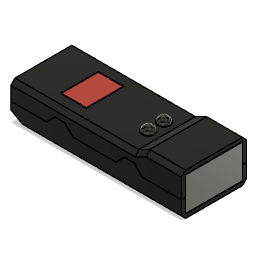
Case-USBtinyISP (Autodesk Fusion 360 design; units mm, degrees)
Autodesk Fusion 360 part; units mm, degrees
note: some values were not read from the file. Chosen so that the rebuilt part matches the saved one: which face or edge a step refers to; which pieces of a blend or face edit are solid. Set by a fixed rule: which sketch regions a step uses.
sketch "Skizze1" plane through (0, 0, 0) normal (0, 1, 0) x (1, 0, 0)
  line L0 (1, 0) -> (35.6, 0)
  line L1 (35.6, 0) -> (35.6, -15.2)
  line L2 (35.6, -15.2) -> (1, -15.2)
  line L3 (0, -14.2) -> (0, -1)
  arc A0 (1, 0) -> (0, -1) centre (1, -1) ccw
  arc A1 (0, -14.2) -> (1, -15.2) centre (1, -14.2) ccw
  line L4 (8.04, -3.725) -> (-1.46, -3.725)
  line L5 (-1.46, -3.725) -> (-1.46, -11.475)
  line L6 (-1.46, -11.475) -> (8.04, -11.475)
  line L7 (8.04, -11.475) -> (8.04, -3.725)
  line L8 (8.04, -3.725) -> (-1.46, -11.475) construction
  line L9 (-1.46, -3.725) -> (8.04, -11.475) construction
  line L10 (35.6, -7.6) -> (40.1, -7.6) construction
  line L11 (35.6, 0.02) -> (44.6, 0.02)
  line L12 (44.6, 0.02) -> (44.6, -15.22)
  line L13 (44.6, -15.22) -> (35.6, -15.22)
  line L14 (35.6, -15.22) -> (35.6, 0.02)
  line L15 (35.6, 0.02) -> (44.6, -15.22) construction
  line L16 (44.6, 0.02) -> (35.6, -15.22) construction
  line L17 (0, -7.6) -> (12, -7.6) construction
  line L18 (15.35, -2.65) -> (8.65, -2.65)
  line L19 (8.65, -2.65) -> (8.65, -12.55)
  line L20 (8.65, -12.55) -> (15.35, -12.55)
  line L21 (15.35, -12.55) -> (15.35, -2.65)
  line L22 (15.35, -2.65) -> (8.65, -12.55) construction
  line L23 (8.65, -2.65) -> (15.35, -12.55) construction
  line L24 (0, -7.6) -> (29.1, -7.6) construction
  line L25 (29.1, -7.6) -> (29.1, -5.5) construction
  line L26 (29.1, -7.6) -> (29.1, -9.7) construction
  line L27 (29.5, -6.1) -> (28.7, -6.1)
  line L28 (28.7, -6.1) -> (28.7, -4.9)
  line L29 (28.7, -4.9) -> (29.5, -4.9)
  line L30 (29.5, -4.9) -> (29.5, -6.1)
  line L31 (29.5, -6.1) -> (28.7, -4.9) construction
  line L32 (28.7, -6.1) -> (29.5, -4.9) construction
  line L33 (29.5, -10.3) -> (28.7, -10.3)
  line L34 (28.7, -10.3) -> (28.7, -9.1)
  line L35 (28.7, -9.1) -> (29.5, -9.1)
  line L36 (29.5, -9.1) -> (29.5, -10.3)
  line L37 (29.5, -10.3) -> (28.7, -9.1) construction
  line L38 (28.7, -10.3) -> (29.5, -9.1) construction
  point P0 (0, -15.2)
  point P1 (3.29, -7.6)
  point P2 (40.1, -7.6)
  point P3 (12, -7.6)
  point P4 (29.1, -5.5)
  point P5 (29.1, -9.7)
  dimension "d4" = 35.6
  dimension "d5" = 15.2
  dimension "d6" = 1
  dimension "d7" = 1
  dimension "d14" = 9.5
  dimension "d15" = 7.75
  dimension "d21" = 4.5
  dimension "d22" = 15.24
  dimension "d23" = 9
  dimension "d28" = 12
  dimension "d29" = 6.7
  dimension "d30" = 9.9
  dimension "d143" = 29.1
  dimension "d144" = 2.1
  dimension "d145" = 2.1
  dimension "d146" = 1.2
  dimension "d147" = 0.8
  dimension "d148" = 1.2
  dimension "d149" = 0.8
  dimension "d261" = 3.29
  constraint horizontal L0
  constraint vertical L1
  constraint horizontal L2
  constraint vertical L3
  constraint coincident origin L3
  constraint coincident origin L0
  constraint tangent L3 A0
  constraint tangent L0 A0
  constraint coincident P0 L2
  constraint coincident P0 L3
  constraint tangent L2 A1
  constraint tangent L3 A1
  constraint midpoint L3 L17.start
  constraint perpendicular L4 L5
  constraint parallel L4 L6
  constraint parallel L5 L7
  constraint horizontal L4
  constraint coincident L8 P1
  constraint coincident L9 P1
  constraint midpoint L1 L10.start
  constraint horizontal L10
  constraint perpendicular L11 L12
  constraint parallel L11 L13
  constraint parallel L12 L14
  constraint horizontal L11
  constraint coincident L15 P2
  constraint coincident L16 P2
  constraint coincident P2 L10.end
  constraint perpendicular L18 L19
  constraint parallel L18 L20
  constraint parallel L19 L21
  constraint horizontal L18
  constraint coincident L22 P3
  constraint coincident L23 P3
  constraint coincident P3 L17.end
  constraint horizontal L17
  constraint horizontal L24
  constraint vertical L26
  constraint vertical L25
  constraint perpendicular L27 L28
  constraint parallel L27 L29
  constraint parallel L28 L30
  constraint horizontal L27
  constraint coincident L31 P4
  constraint coincident L32 P4
  constraint coincident P4 L25.end
  constraint perpendicular L33 L34
  constraint parallel L33 L35
  constraint parallel L34 L36
  constraint horizontal L33
  constraint coincident L37 P5
  constraint coincident L38 P5
  constraint coincident P5 L26.end
  constraint coincident P1 L17
  measures "d4" distance of origin L0.end
  measures "d5" distance of origin P0
  measures "d6" radius of A0
  measures "d7" radius of A1
  measures "d14" distance of L5.end L6.end
  measures "d15" distance of L4.end L5.end
  measures "d21" distance of L10.start P2
  measures "d22" distance of L11.end L12.end
  measures "d23" distance of L12.end L13.end
  measures "d28" distance of L17.start P3
  measures "d29" distance of L19.end L20.end
  measures "d30" distance of L18.end L19.end
  measures "d143" distance of L17.start L24.end
  measures "d144" distance of L24.end P4
  measures "d145" distance of L24.end P5
  measures "d146" distance of L27.end L28.end
  measures "d147" distance of L28.end L29.end
  measures "d148" distance of L33.end L34.end
  measures "d149" distance of L34.end L35.end
  measures "d261" distance of L17.start P1
sketch "Skizze2" plane through (0, 0, 0) normal (0, 1, 0) x (1, 0, 0)
  line L0 (15.45, -12.65) -> (8.55, -12.65)
  line L1 (8.55, -12.65) -> (8.55, -2.55)
  line L2 (8.55, -2.55) -> (15.45, -2.55)
  line L3 (15.45, -2.55) -> (15.45, -12.65)
  line L4 (15.45, -12.65) -> (8.55, -2.55) construction
  line L5 (8.55, -12.65) -> (15.45, -2.55) construction
  line L6 (0, 0) -> (-0.1, 0) construction
  line L7 (-0.1, 0) -> (-0.1, 0.1) construction
  line L8 (1, 0.1) -> (44.6, 0.1)
  line L9 (44.6, 0.1) -> (44.6, -15.3)
  line L10 (44.6, -15.3) -> (1, -15.3)
  line L11 (-0.1, -14.2) -> (-0.1, -1)
  arc A0 (1, 0.1) -> (-0.1, -1) centre (1, -1) ccw
  arc A1 (-0.1, -14.2) -> (1, -15.3) centre (1, -14.2) ccw
  line L12 (-0.1, 0.1) -> (-1.1, 0.1) construction
  line L13 (-1.1, 0.1) -> (-1.1, 1.1) construction
  line L14 (1, 1.1) -> (44.6, 1.1)
  line L15 (44.6, 1.1) -> (44.6, -16.3)
  line L16 (44.6, -16.3) -> (1, -16.3)
  line L17 (-1.1, -14.2) -> (-1.1, -1)
  arc A2 (1, 1.1) -> (-1.1, -1) centre (1, -1) ccw
  arc A3 (-1.1, -14.2) -> (1, -16.3) centre (1, -14.2) ccw
  line L18 (-0.1, -7.6) -> (-0.6, -7.6) construction
  line L19 (-0.1, -3.625) -> (-1.1, -3.625)
  line L20 (-1.1, -3.625) -> (-1.1, -11.575)
  line L21 (-1.1, -11.575) -> (-0.1, -11.575)
  line L22 (-0.1, -11.575) -> (-0.1, -3.625)
  line L23 (-0.1, -3.625) -> (-1.1, -11.575) construction
  line L24 (-1.1, -3.625) -> (-0.1, -11.575) construction
  line L25 (-1.1, 1.1) -> (44.6, 1.1)
  line L26 (44.6, 1.1) -> (44.6, -16.3)
  line L27 (44.6, -16.3) -> (-1.1, -16.3)
  line L28 (-1.1, -16.3) -> (-1.1, 1.1)
  line L29 (-0.1, 0.1) -> (44.6, 0.1)
  line L30 (44.6, 0.1) -> (44.6, -15.3)
  line L31 (44.6, -15.3) -> (-0.1, -15.3)
  line L32 (-0.1, -15.3) -> (-0.1, 0.1)
  line L33 (12, -7.6) -> (35, -7.6) construction
  line L34 (35, -7.6) -> (35, 1.1)
  line L35 (35, -7.6) -> (35, -16.3)
  line L36 (35, -7.6) -> (35.2361, -7.6) construction
  line L37 (35.2361, -7.6) -> (35.2361, 1.1)
  line L38 (35.2361, -7.6) -> (35.2361, -16.3)
  circle A4 centre (29.1, -5.5) radius 1.6
  circle A5 centre (29.1, -5.5) radius 1.4
  circle A6 centre (29.1, -9.7) radius 1.4
  circle A7 centre (29.1, -9.7) radius 1.6
  line L39 (-0.1, -15.3) -> (-0.1, -15.8) construction
  line L40 (-0.1, -15.8) -> (12, -15.8) construction
  line L41 (13.25, -16.3) -> (10.75, -16.3)
  line L42 (10.75, -16.3) -> (10.75, -15.3)
  line L43 (10.75, -15.3) -> (13.25, -15.3)
  line L44 (13.25, -15.3) -> (13.25, -16.3)
  line L45 (13.25, -16.3) -> (10.75, -15.3) construction
  line L46 (10.75, -16.3) -> (13.25, -15.3) construction
  line L47 (12, -15.8) -> (12, -15.05) construction
  line L48 (12, -15.05) -> (12, -14.5) construction
  line L49 (13.25, -15.3) -> (10.75, -15.3)
  line L50 (10.75, -15.3) -> (10.75, -14.8)
  line L51 (10.75, -14.8) -> (13.25, -14.8)
  line L52 (13.25, -14.8) -> (13.25, -15.3)
  line L53 (13.25, -15.3) -> (10.75, -14.8) construction
  line L54 (10.75, -15.3) -> (13.25, -14.8) construction
  line L55 (13.7056, -15.3) -> (10.2944, -15.3)
  line L56 (10.2944, -15.3) -> (10.2944, -13.7)
  line L57 (10.2944, -13.7) -> (13.7056, -13.7)
  line L58 (13.7056, -13.7) -> (13.7056, -15.3)
  line L59 (13.7056, -15.3) -> (10.2944, -13.7) construction
  line L60 (10.2944, -15.3) -> (13.7056, -13.7) construction
  line L61 (13.3914, -16.3) -> (10.6086, -16.3)
  line L62 (10.6086, -16.3) -> (10.6086, -15.3)
  line L63 (10.6086, -15.3) -> (13.3914, -15.3)
  line L64 (13.3914, -15.3) -> (13.3914, -16.3)
  line L65 (13.3914, -16.3) -> (10.6086, -15.3) construction
  line L66 (10.6086, -16.3) -> (13.3914, -15.3) construction
  line L67 (12, -15.05) -> (12, -15) construction
  line L68 (13.2914, -15.3) -> (10.7086, -15.3)
  line L69 (10.7086, -15.3) -> (10.7086, -14.7)
  line L70 (10.7086, -14.7) -> (13.2914, -14.7)
  line L71 (13.2914, -14.7) -> (13.2914, -15.3)
  line L72 (13.2914, -15.3) -> (10.7086, -14.7) construction
  line L73 (10.7086, -15.3) -> (13.2914, -14.7) construction
  line L74 (12, -15.8) -> (21.3016, -15.8) construction
  line L75 (21.3016, -15.8) -> (21.3016, 0.6) construction
  line L76 (31.8532, -16.3) -> (31.8532, -15.3)
  line L77 (31.9946, -16.3) -> (31.9946, -15.3)
  line L78 (31.8946, -15.3) -> (31.8946, -14.7)
  line L79 (31.8532, -15.3) -> (31.8532, -14.8)
  line L80 (31.8532, -14.8) -> (29.3532, -14.8)
  line L81 (31.8946, -14.7) -> (29.3118, -14.7)
  line L82 (29.3532, -15.3) -> (29.3532, -16.3)
  line L83 (29.2118, -15.3) -> (29.2118, -16.3)
  line L84 (29.3532, -14.8) -> (29.3532, -15.3)
  line L85 (29.3118, -14.7) -> (29.3118, -15.3)
  line L86 (28.8976, -13.7) -> (28.8976, -15.3)
  line L87 (32.3089, -13.7) -> (28.8976, -13.7)
  line L88 (32.3089, -15.3) -> (32.3089, -13.7)
  line L89 (10.75, 0.1) -> (10.75, -0.4)
  line L90 (10.75, -0.4) -> (13.25, -0.4)
  line L91 (10.7086, -0.5) -> (13.2914, -0.5)
  line L92 (10.7086, 0.1) -> (10.7086, -0.5)
  line L93 (13.2914, -0.5) -> (13.2914, 0.1)
  line L94 (13.25, -0.4) -> (13.25, 0.1)
  line L95 (13.25, 0.1) -> (13.25, 1.1)
  line L96 (13.3914, 0.1) -> (13.3914, 1.1)
  line L97 (10.6086, 1.1) -> (10.6086, 0.1)
  line L98 (10.75, 1.1) -> (10.75, 0.1)
  line L99 (10.2944, 0.1) -> (10.2944, -1.5)
  line L100 (10.2944, -1.5) -> (13.7056, -1.5)
  line L101 (13.7056, -1.5) -> (13.7056, 0.1)
  line L102 (29.3532, -0.4) -> (29.3532, 0.1)
  line L103 (29.3118, -0.5) -> (29.3118, 0.1)
  line L104 (31.8532, -0.4) -> (29.3532, -0.4)
  line L105 (31.8946, -0.5) -> (29.3118, -0.5)
  line L106 (28.8976, -1.5) -> (28.8976, 0.1)
  line L107 (32.3089, -1.5) -> (28.8976, -1.5)
  line L108 (29.2118, 0.1) -> (29.2118, 1.1)
  line L109 (29.3532, 0.1) -> (29.3532, 1.1)
  line L110 (31.9946, 1.1) -> (31.9946, 0.1)
  line L111 (31.8532, 1.1) -> (31.8532, 0.1)
  line L112 (31.8532, 0.1) -> (31.8532, -0.4)
  line L113 (31.8946, 0.1) -> (31.8946, -0.5)
  line L114 (32.3089, 0.1) -> (32.3089, -1.5)
  line L115 (12, -15) -> (12, -14.95) construction
  line L116 (10.7086, -14.7) -> (13.2914, -14.7)
  line L117 (13.2914, -14.7) -> (13.2914, -15.2)
  line L118 (13.2914, -15.2) -> (10.7086, -15.2)
  line L119 (10.7086, -15.2) -> (10.7086, -14.7)
  line L120 (10.7086, -14.7) -> (13.2914, -15.2) construction
  line L121 (13.2914, -14.7) -> (10.7086, -15.2) construction
  line L122 (29.3118, -15.2) -> (31.8946, -15.2)
  line L123 (13.2914, 0) -> (10.7086, 0)
  line L124 (29.3118, 0) -> (31.8946, 0)
  line L125 (12, -14.95) -> (12, -14.75) construction
  line L126 (7.3672, -15.3) -> (16.6328, -15.3)
  line L127 (16.6328, -15.3) -> (16.6328, -14.2)
  line L128 (16.6328, -14.2) -> (7.3672, -14.2)
  line L129 (7.3672, -14.2) -> (7.3672, -15.3)
  line L130 (7.3672, -15.3) -> (16.6328, -14.2) construction
  line L131 (16.6328, -15.3) -> (7.3672, -14.2) construction
  line L132 (25.9704, -14.2) -> (35.2361, -14.2)
  line L133 (25.9704, -15.3) -> (25.9704, -14.2)
  line L134 (35.2361, -14.2) -> (35.2361, -15.3)
  line L135 (16.6328, -1) -> (7.3672, -1)
  line L136 (16.6328, 0.1) -> (16.6328, -1)
  line L137 (7.3672, -1) -> (7.3672, 0.1)
  line L138 (25.9704, 0.1) -> (25.9704, -1)
  line L139 (25.9704, -1) -> (35.2361, -1)
  line L140 (35.2361, -1) -> (35.2361, 0.1)
  line L141 (12, -15.8) -> (12, -15.25) construction
  line L142 (10.6086, -15.3) -> (13.3914, -15.3)
  line L143 (13.3914, -15.3) -> (13.3914, -15.2)
  line L144 (13.3914, -15.2) -> (10.6086, -15.2)
  line L145 (10.6086, -15.2) -> (10.6086, -15.3)
  line L146 (10.6086, -15.3) -> (13.3914, -15.2) construction
  line L147 (13.3914, -15.3) -> (10.6086, -15.2) construction
  line L148 (29.2118, -15.3) -> (29.2118, -15.2)
  line L149 (29.2118, -15.2) -> (31.9946, -15.2)
  line L150 (31.9946, -15.2) -> (31.9946, -15.3)
  line L151 (29.2118, 0) -> (31.9946, 0)
  line L152 (29.2118, 0.1) -> (29.2118, 0)
  line L153 (31.9946, 0) -> (31.9946, 0.1)
  line L154 (13.3914, 0.1) -> (13.3914, 0)
  line L155 (13.3914, 0) -> (10.6086, 0)
  line L156 (10.6086, 0) -> (10.6086, 0.1)
  point P0 (12, -7.6)
  point P1 (12, -7.6)
  point P2 (-0.1, -15.3)
  point P3 (-1.1, -16.3)
  point P4 (-0.6, -7.6)
  point P5 (12, -7.6)
  point P6 (29.1, -5.5)
  point P7 (29.1, -9.7)
  point P8 (12, -15.8)
  point P9 (12, -15.05)
  point P10 (12, -14.5)
  point P11 (12, -15.8)
  point P12 (12, -15)
  point P13 (12, -14.95)
  point P14 (12, -14.75)
  point P15 (12, -15.25)
  dimension "d31" = 6.9
  dimension "d32" = 10.1
  dimension "d34" = 0.1
  dimension "d35" = 0.1
  dimension "d36" = 15.4
  dimension "d37" = 44.7
  dimension "d38" = 1.1
  dimension "d39" = 1.1
  dimension "d40" = 1
  dimension "d41" = 1
  dimension "d42" = 45.7
  dimension "d43" = 17.4
  dimension "d44" = 2.1
  dimension "d45" = 2.1
  dimension "d46" = 0.5
  dimension "d47" = 7.95
  dimension "d48" = 1
  dimension "d82" = 45.7
  dimension "d83" = 17.4
  dimension "d84" = 15.4
  dimension "d85" = 44.7
  dimension "d105" = 23
  dimension "d106" = 8.7
  dimension "d107" = 8.7
  dimension "d114" = 0.2361
  dimension "d115" = 8.7
  dimension "d116" = 8.7
  dimension "d151" = 3.2
  dimension "d152" = 2.8
  dimension "d153" = 2.8
  dimension "d154" = 3.2
  dimension "d182" = 0.5
  dimension "d183" = 12.1
  dimension "d189" = 2.5
  dimension "d190" = 1
  dimension "d193" = 0.75
  dimension "d194" = 0.55
  dimension "d195" = 2.5
  dimension "d196" = 0.5
  dimension "d197" = 3.4113
  dimension "d198" = 1.6
  dimension "d199" = 2.7828
  dimension "d200" = 1
  dimension "d201" = 0.05
  dimension "d202" = 2.5828
  dimension "d203" = 0.6
  dimension "d205" = 16.4
  dimension "d206" = 0.05
  dimension "d207" = 0.5
  dimension "d208" = 2.5828
  dimension "d224" = 0.2
  dimension "d225" = 9.2657
  dimension "d226" = 1.1
  dimension "d240" = 0.55
  dimension "d241" = 2.7828
  dimension "d242" = 0.1
  constraint perpendicular L0 L1
  constraint parallel L0 L2
  constraint parallel L1 L3
  constraint horizontal L0
  constraint coincident L4 P1
  constraint coincident L5 P1
  constraint coincident P1 P0
  constraint coincident L6.start origin
  constraint horizontal L8
  constraint vertical L9
  constraint horizontal L10
  constraint vertical L11
  constraint coincident L7.end L8
  constraint coincident L7.end L11
  constraint tangent L8 A0
  constraint tangent L11 A0
  constraint coincident P2 L10
  constraint coincident P2 L11
  constraint tangent L10 A1
  constraint tangent L11 A1
  constraint horizontal L12
  constraint vertical L13
  constraint horizontal L6
  constraint vertical L7
  constraint horizontal L14
  constraint vertical L15
  constraint horizontal L16
  constraint vertical L17
  constraint coincident L13.end L14
  constraint coincident L13.end L17
  constraint tangent L14 A2
  constraint tangent L17 A2
  constraint coincident P3 L16
  constraint coincident P3 L17
  constraint tangent L16 A3
  constraint tangent L17 A3
  constraint midpoint L11 L18.start
  constraint perpendicular L19 L20
  constraint parallel L19 L21
  constraint parallel L20 L22
  constraint horizontal L19
  constraint coincident L23 P4
  constraint coincident L24 P4
  constraint coincident P4 L18.end
  constraint horizontal L18
  constraint horizontal L25
  constraint vertical L26
  constraint horizontal L27
  constraint vertical L28
  constraint horizontal L29
  constraint vertical L30
  constraint horizontal L31
  constraint vertical L32
  constraint coincident P5 P1
  constraint horizontal L33
  constraint vertical L35
  constraint vertical L34
  constraint vertical L37
  constraint vertical L38
  constraint coincident P6 A4.centre
  constraint coincident P7 A6.centre
  constraint horizontal L40
  constraint vertical L39
  constraint perpendicular L41 L42
  constraint parallel L41 L43
  constraint parallel L42 L44
  constraint horizontal L41
  constraint coincident L45 P11
  constraint coincident L46 P11
  constraint coincident P11 P8
  constraint vertical L47
  constraint vertical L48
  constraint perpendicular L49 L50
  constraint parallel L49 L51
  constraint parallel L50 L52
  constraint horizontal L49
  constraint coincident L53 P9
  constraint coincident L54 P9
  constraint coincident P9 L47.end
  constraint perpendicular L55 L56
  constraint parallel L55 L57
  constraint parallel L56 L58
  constraint horizontal L55
  constraint coincident L59 P10
  constraint coincident L60 P10
  constraint coincident P10 L48.end
  constraint perpendicular L61 L62
  constraint parallel L61 L63
  constraint parallel L62 L64
  constraint horizontal L61
  constraint coincident L65 P11
  constraint coincident L66 P11
  constraint vertical L67
  constraint perpendicular L68 L69
  constraint parallel L68 L70
  constraint parallel L69 L71
  constraint horizontal L68
  constraint coincident L72 P12
  constraint coincident L73 P12
  constraint coincident P12 L67.end
  constraint horizontal L74
  constraint vertical L75
  constraint symmetric L41.start L75 L82.end
  constraint symmetric L41.end L75 L76.start
  constraint symmetric L42.end L75 L76.end
  constraint symmetric L43.end L75 L82.start
  constraint symmetric L50.end L75 L79.end
  constraint symmetric L51.end L75 L80.end
  constraint symmetric L55.start L75 L86.end
  constraint symmetric L55.end L75 L88.start
  constraint symmetric L56.end L75 L87.start
  constraint symmetric L57.end L75 L86.start
  constraint symmetric L61.start L75 L83.end
  constraint symmetric L61.end L75 L77.start
  constraint symmetric L62.end L75 L77.end
  constraint symmetric L63.end L75 L83.start
  constraint symmetric L68.start L75 L85.end
  constraint symmetric L68.end L75 L78.start
  constraint symmetric L69.end L75 L78.end
  constraint symmetric L70.end L75 L81.end
  constraint symmetric L33 L41.start L95.end
  constraint symmetric L33 L41.end L98.start
  constraint symmetric L33 L42.end L89.start
  constraint symmetric L33 L43.end L94.end
  constraint symmetric L33 L50.end L89.end
  constraint symmetric L33 L51.end L90.end
  constraint symmetric L33 L55.start L101.end
  constraint symmetric L33 L55.end L99.start
  constraint symmetric L33 L56.end L99.end
  constraint symmetric L33 L57.end L100.end
  constraint symmetric L33 L61.start L96.end
  constraint symmetric L33 L61.end L97.start
  constraint symmetric L33 L62.end L97.end
  constraint symmetric L33 L63.end L96.start
  constraint symmetric L33 L68.start L93.end
  constraint symmetric L33 L68.end L92.start
  constraint symmetric L33 L69.end L91.start
  constraint symmetric L33 L70.end L91.end
  constraint symmetric L33 L76.start L111.start
  constraint symmetric L33 L76.end L111.end
  constraint symmetric L33 L77.start L110.start
  constraint symmetric L33 L77.end L110.end
  constraint symmetric L33 L78.start L113.start
  constraint symmetric L33 L78.end L105.start
  constraint symmetric L33 L79.end L104.start
  constraint symmetric L33 L80.end L102.start
  constraint symmetric L33 L81.end L103.start
  constraint symmetric L33 L82.start L102.end
  constraint symmetric L33 L82.end L109.end
  constraint symmetric L33 L83.start L108.start
  constraint symmetric L33 L83.end L108.end
  constraint symmetric L33 L85.end L103.end
  constraint symmetric L33 L86.start L106.start
  constraint symmetric L33 L86.end L106.end
  constraint symmetric L33 L87.start L107.start
  constraint symmetric L33 L88.start L114.start
  constraint vertical L115
  constraint perpendicular L116 L117
  constraint parallel L116 L118
  constraint parallel L117 L119
  constraint horizontal L116
  constraint coincident L120 P13
  constraint coincident L121 P13
  constraint coincident P13 L115.end
  constraint symmetric L75 L117.end L122.start
  constraint symmetric L75 L118.end L122.end
  constraint symmetric L33 L117.end L123.start
  constraint symmetric L33 L118.end L123.end
  constraint symmetric L33 L122.start L124.start
  constraint symmetric L33 L122.end L124.end
  constraint vertical L125
  constraint perpendicular L126 L127
  constraint parallel L126 L128
  constraint parallel L127 L129
  constraint horizontal L126
  constraint coincident L130 P14
  constraint coincident L131 P14
  constraint coincident P14 L125.end
  constraint symmetric L75 L126.start L134.end
  constraint symmetric L75 L126.end L133.start
  constraint symmetric L75 L127.end L132.start
  constraint symmetric L75 L128.end L132.end
  constraint symmetric L33 L126.start L137.end
  constraint symmetric L33 L126.end L136.start
  constraint symmetric L33 L127.end L135.start
  constraint symmetric L33 L128.end L135.end
  constraint symmetric L33 L132.start L138.end
  constraint symmetric L33 L132.end L139.end
  constraint symmetric L33 L133.start L138.start
  constraint symmetric L33 L134.end L140.end
  constraint vertical L141
  constraint perpendicular L142 L143
  constraint parallel L142 L144
  constraint parallel L143 L145
  constraint horizontal L142
  constraint coincident L146 P15
  constraint coincident L147 P15
  constraint coincident P15 L141.end
  constraint symmetric L75 L62.end L77.end
  constraint symmetric L75 L63.end L83.start
  constraint symmetric L75 L143.end L148.end
  constraint symmetric L75 L144.end L149.end
  constraint symmetric L33 L143.end L154.end
  constraint symmetric L33 L144.end L155.end
  constraint symmetric L33 L148.end L151.start
  constraint symmetric L33 L149.end L151.end
  constraint coincident L37 L140.end
  measures "d31" distance of L1.end L2.end
  measures "d32" distance of L0.end L1.end
  measures "d34" distance of L6.start L6.end
  measures "d35" distance of L6.end L7.end
  measures "d36" distance of L7.end P2
  measures "d37" distance of L7.end L8.end
  measures "d38" radius of A0
  measures "d39" radius of A1
  measures "d40" distance of L7.end L12.end
  measures "d41" distance of L12.end L13.end
  measures "d42" distance of L13.end L14.end
  measures "d43" distance of L13.end P3
  measures "d44" radius of A2
  measures "d45" radius of A3
  measures "d46" distance of L18.start P4
  measures "d47" distance of L19.end L20.end
  measures "d48" distance of L20.end L21.end
  measures "d82" distance of L13.end L14.end
  measures "d83" distance of L13.end P3
  measures "d84" distance of L7.end P2
  measures "d85" distance of L7.end L8.end
  measures "d105" distance of P5 L33.end
  measures "d106" distance of L33.end L34.end
  measures "d107" distance of L33.end L35.end
  measures "d114" distance of L33.end L36.end
  measures "d115" distance of L36.end L37.end
  measures "d116" distance of L36.end L38.end
  measures "d151" diameter of A4
  measures "d152" diameter of A5
  measures "d153" diameter of A6
  measures "d154" diameter of A7
  measures "d182" distance of P2 L39.end
  measures "d183" distance of L39.end P11
  measures "d189" distance of L42.end L43.end
  measures "d190" distance of L41.end L42.end
  measures "d193" distance of P11 P9
  measures "d194" distance of P9 P10
  measures "d195" distance of L50.end L51.end
  measures "d196" distance of L42.end L50.end
  measures "d197" distance of L56.end L57.end
  measures "d198" distance of L55.end L56.end
  measures "d199" distance of L62.end L63.end
  measures "d200" distance of L61.end L62.end
  measures "d201" distance of P9 P12
  measures "d202" distance of L69.end L70.end
  measures "d203" distance of L68.end L69.end
  measures "d205" distance of L74.end L75.end
  measures "d206" distance of P12 P13
  measures "d207" distance of L70.end L117.end
  measures "d208" distance of L117.end L118.end
  measures "d224" distance of P13 P14
  measures "d225" distance of L127.end L128.end
  measures "d226" distance of L126.end L127.end
  measures "d240" distance of P11 P15
  measures "d241" distance of L143.end L144.end
  measures "d242" distance of L63.end L143.end
extrude "Extrusion1" add sketch "Skizze1" along normal blind 1.6 contours L0 L1 L2 L3 A0 A1 L4 L6 L7 L14 | L3 L4 L6 L7 | L18 L19 L20 L21 | L27 L28 L29 L30 | L33 L34 L35 L36 makes body 1
extrude "Extrusion2" add sketch "Skizze1" along normal blind 4.5 from surface at 1.6 separate body contours L3 L4 L6 L7 | L3 L4 L5 L6 makes body 2
extrude "Extrusion3" cut sketch "Skizze1" along normal blind 1.6 contours L3 L4 L6 L7 bodies 2
extrude "Extrusion4" add sketch "Skizze1" along normal blind 7.69 and the other way blind 1.31 separate body contours L1 L11 L12 L13 L14 makes body 3
extrude "Extrusion5" add sketch "Skizze1" along normal blind 5.7 from surface at 1.6 separate body contours L18 L19 L20 L21 makes body 4
extrude "Extrusion16" add sketch "Skizze1" along normal blind 0.6 from surface at 1.6 separate body contours L27 L28 L29 L30 | L33 L34 L35 L36 makes body 5 at (28.9667, 1.6, 5.3) makes body 6 at (28.9667, 1.6, 9.5)
extrude "Extrusion17" add sketch "Skizze2" along normal blind 5 from surface at 2.3 separate body contours A5 | A6 makes body 7 at (30.4983, 5.6333, 9.7698) makes body 8 at (30.4983, 5.6333, 5.5698)
extrude "Extrusion18" add sketch "Skizze2" along normal blind 1.6 from surface at 7.3 contours A4 | A5 | A6 | A7 bodies 7 8
fillet "Abrundung5" radius 1.6 2 edges at (27.6083, 8.9, 10.2786) (27.6083, 8.9, 6.0786) on bodies 7 8
extrude "Extrusion6" add sketch "Skizze2" along normal blind 1 from surface at -2.41 separate body contours L0 L1 L2 L3 | L8 L11 L14 L17 A2 L19 L25 L28 L29 L32 L97 | L8 L10 L11 A0 A1 L22 L29 L31 L32 L34 L35 L56 L57 L58 L86 L87 L88 L99 L100 L101 L106 L107 L114 L127 L128 L129 L132 L133 L135 L136 L137 L138 L139 | A0 L29 L32 | L8 L29 L99 L135 L137 | L8 L29 L91 L92 L93 L99 L101 L135 L154 L155 L156 | L11 L17 L19 L20 L21 L22 L28 L32 | L8 L14 L25 L29 L97 L98 | L8 L29 L92 L155 L156 | L99 L100 L101 L135 | L10 L11 L16 L17 A3 L21 L27 L28 L31 L32 L55 L62 L126 | L8 L29 L89 L92 L123 L155 | L8 L29 L101 L135 L136 | A1 L31 L32 | A2 L25 L28 | L8 L14 L25 L29 L95 L98 | L8 L29 L89 L94 L123 L155 | L89 L90 L91 L92 L93 L94 L123 L155 | L8 L14 L25 L29 L96 L108 | A3 L27 L28 | L8 L14 L25 L29 L95 L96 | L8 L29 L93 L94 L123 L155 | L89 L90 L94 L123 L155 | L8 L29 L93 L154 L155 | L10 L31 L56 L126 L128 L129 | L8 L29 L106 L138 L139 | L10 L31 L55 L56 L58 L69 L70 L71 L116 L117 L119 L126 L128 L143 L144 L145 | L10 L16 L27 L31 L42 L55 L61 L62 L63 L68 L126 L142 | L8 L14 L25 L29 L108 L109 | L8 L29 L103 L105 L106 L113 L114 L139 L151 L152 L153 | L10 L31 L55 L63 L69 L126 L142 L144 L145 | L56 L57 L58 L128 | L10 L16 L27 L31 L41 L42 L43 L44 L49 L55 L61 L63 L68 L126 L142 | L8 L14 L25 L29 L109 L111 | L8 L29 L103 L151 L152 | L106 L107 L114 L139 | L10 L31 L50 L55 L63 L68 L69 L118 L126 L142 L144 | L10 L31 L58 L126 L127 L128 | L10 L16 L27 L31 L44 L55 L61 L63 L64 L68 L126 L142 | L10 L31 L43 L49 L50 L52 L55 L63 L68 L118 L126 L142 L144 | L8 L14 L25 L29 L110 L111 | L8 L29 L102 L103 L124 L151 | L8 L29 L102 L112 L124 L151 | L8 L29 L34 L114 L139 | L50 L51 L52 L69 L70 L71 L116 L117 L118 L119 L144 | L10 L16 L27 L31 L55 L64 L83 L126 | L10 L31 L52 L55 L63 L68 L71 L118 L126 L142 L144 | L50 L51 L52 L118 L144 | L8 L14 L25 L29 L34 L110 | L8 L29 L112 L113 L124 L151 | L102 L104 L112 L124 L151 | L102 L103 L104 L105 L112 L113 L124 L151 | L34 L35 L37 L38 L132 L139 | L8 L29 L34 L37 L139 L140 | L10 L31 L55 L63 L71 L126 L142 L143 L144 | L10 L16 L27 L31 L82 L83 | L8 L14 L25 L29 L34 L37 | L8 L29 L113 L151 L153 | L8 L9 L10 L15 L26 L29 L30 L31 L37 L38 L134 L140 | L10 L31 L86 L132 L133 | L10 L16 L27 L31 L76 L82 | L10 L31 L85 L148 L149 | L10 L31 L78 L81 L85 L86 L88 L132 L148 L149 L150 | L8 L14 L15 L25 L26 L29 L37 | L10 L31 L35 L38 L132 L134 | L10 L31 L35 L88 L132 | L10 L16 L27 L31 L76 L77 | L10 L31 L79 L84 L122 L149 | L10 L31 L84 L85 L122 L149 | L10 L16 L27 L31 L35 L77 | L10 L16 L27 L31 L35 L38 | L86 L87 L88 L132 | L10 L31 L78 L79 L122 L149 | L78 L79 L80 L81 L84 L85 L122 L149 | L79 L80 L84 L122 L149 | L10 L15 L16 L26 L27 L31 L38 | L10 L31 L78 L149 L150 | A4 | A5 | A6 | A7 makes body 9
extrude "Extrusion7" add sketch "Skizze2" along normal blind 3.855 from surface at -1.41 contours L8 L11 L14 L17 A2 L19 L25 L28 L29 L32 L97 | L8 L14 L25 L29 L97 L98 | L10 L11 L16 L17 A3 L21 L27 L28 L31 L32 L55 L62 L126 | A2 L25 L28 | L8 L14 L25 L29 L95 L98 | L8 L14 L25 L29 L96 L108 | A3 L27 L28 | L8 L14 L25 L29 L95 L96 | L10 L16 L27 L31 L42 L55 L61 L62 L63 L68 L126 L142 | L8 L14 L25 L29 L108 L109 | L10 L16 L27 L31 L41 L42 L43 L44 L49 L55 L61 L63 L68 L126 L142 | L8 L14 L25 L29 L109 L111 | L10 L16 L27 L31 L44 L55 L61 L63 L64 L68 L126 L142 | L8 L14 L25 L29 L110 L111 | L10 L16 L27 L31 L55 L64 L83 L126 | L8 L14 L25 L29 L34 L110 | L10 L16 L27 L31 L82 L83 | L8 L14 L25 L29 L34 L37 | L10 L16 L27 L31 L76 L82 | L8 L14 L15 L25 L26 L29 L37 | L10 L16 L27 L31 L76 L77 | L10 L16 L27 L31 L35 L77 | L10 L16 L27 L31 L35 L38 | L10 L15 L16 L26 L27 L31 L38 bodies 9
extrude "Extrusion8" add sketch "Skizze2" along normal blind -1.41 and the other way blind -1.5 contours L11 L17 L19 L20 L21 L22 L28 L32 bodies 9
extrude "Extrusion9" add sketch "Skizze2" along normal blind 1 from surface at 7.79 separate body contours L34 L35 L37 L38 L132 L139 | L8 L29 L34 L37 L139 L140 | L8 L14 L25 L29 L34 L37 | L8 L9 L10 L15 L26 L29 L30 L31 L37 L38 L134 L140 | L8 L14 L15 L25 L26 L29 L37 | L10 L31 L35 L38 L132 L134 | L10 L16 L27 L31 L35 L38 | L10 L15 L16 L26 L27 L31 L38 makes body 10
extrude "Extrusion15" add sketch "Skizze2" along normal blind 1.49 from surface at 6.3 contours L34 L35 L37 L38 L132 L139 | L8 L29 L34 L37 L139 L140 | L10 L31 L35 L38 L132 L134 bodies 10
extrude "Extrusion10" add sketch "Skizze2" against normal up to surface (5.345 mm away) from surface at 7.79 contours L8 L14 L25 L29 L34 L37 | L8 L14 L15 L25 L26 L29 L37 | L10 L16 L27 L31 L35 L38 | L10 L15 L16 L26 L27 L31 L38 bodies 10
extrude "Extrusion13" add sketch "Skizze2" along normal blind 1 from surface at 6.3 contours L8 L11 L14 L17 A2 L19 L25 L28 L29 L32 L97 | L8 L10 L11 A0 A1 L22 L29 L31 L32 L34 L35 L56 L57 L58 L86 L87 L88 L99 L100 L101 L106 L107 L114 L127 L128 L129 L132 L133 L135 L136 L137 L138 L139 | A0 L29 L32 | L8 L29 L99 L135 L137 | L8 L29 L91 L92 L93 L99 L101 L135 L154 L155 L156 | L11 L17 L19 L20 L21 L22 L28 L32 | L8 L14 L25 L29 L97 L98 | L8 L29 L92 L155 L156 | L99 L100 L101 L135 | L10 L11 L16 L17 A3 L21 L27 L28 L31 L32 L55 L62 L126 | L8 L29 L89 L92 L123 L155 | L8 L29 L101 L135 L136 | A1 L31 L32 | A2 L25 L28 | L8 L14 L25 L29 L95 L98 | L8 L29 L89 L94 L123 L155 | L89 L90 L91 L92 L93 L94 L123 L155 | L8 L14 L25 L29 L96 L108 | A3 L27 L28 | L8 L14 L25 L29 L95 L96 | L8 L29 L93 L94 L123 L155 | L89 L90 L94 L123 L155 | L8 L29 L93 L154 L155 | L10 L31 L56 L126 L128 L129 | L8 L29 L106 L138 L139 | L10 L31 L55 L56 L58 L69 L70 L71 L116 L117 L119 L126 L128 L143 L144 L145 | L10 L16 L27 L31 L42 L55 L61 L62 L63 L68 L126 L142 | L8 L14 L25 L29 L108 L109 | L8 L29 L103 L105 L106 L113 L114 L139 L151 L152 L153 | L10 L31 L55 L63 L69 L126 L142 L144 L145 | L56 L57 L58 L128 | L10 L16 L27 L31 L41 L42 L43 L44 L49 L55 L61 L63 L68 L126 L142 | L8 L14 L25 L29 L109 L111 | L8 L29 L103 L151 L152 | L106 L107 L114 L139 | L10 L31 L50 L55 L63 L68 L69 L118 L126 L142 L144 | L10 L31 L58 L126 L127 L128 | L10 L16 L27 L31 L44 L55 L61 L63 L64 L68 L126 L142 | L10 L31 L43 L49 L50 L52 L55 L63 L68 L118 L126 L142 L144 | L8 L14 L25 L29 L110 L111 | L8 L29 L102 L103 L124 L151 | L8 L29 L102 L112 L124 L151 | L8 L29 L34 L114 L139 | L50 L51 L52 L69 L70 L71 L116 L117 L118 L119 L144 | L10 L16 L27 L31 L55 L64 L83 L126 | L10 L31 L52 L55 L63 L68 L71 L118 L126 L142 L144 | L50 L51 L52 L118 L144 | L8 L14 L25 L29 L34 L110 | L8 L29 L112 L113 L124 L151 | L102 L104 L112 L124 L151 | L102 L103 L104 L105 L112 L113 L124 L151 | L10 L31 L55 L63 L71 L126 L142 L143 L144 | L10 L16 L27 L31 L82 L83 | L8 L29 L113 L151 L153 | L10 L31 L86 L132 L133 | L10 L16 L27 L31 L76 L82 | L10 L31 L85 L148 L149 | L10 L31 L78 L81 L85 L86 L88 L132 L148 L149 L150 | L10 L31 L35 L88 L132 | L10 L16 L27 L31 L76 L77 | L10 L31 L79 L84 L122 L149 | L10 L31 L84 L85 L122 L149 | L10 L16 L27 L31 L35 L77 | L86 L87 L88 L132 | L10 L31 L78 L79 L122 L149 | L78 L79 L80 L81 L84 L85 L122 L149 | L79 L80 L84 L122 L149 | L10 L31 L78 L149 L150 | A4 | A7 bodies 10
extrude "Extrusion14" add sketch "Skizze2" against normal up to surface (3.855 mm away) from surface at 6.3 contours L8 L11 L14 L17 A2 L19 L25 L28 L29 L32 L97 | L8 L29 L99 L135 L137 | L8 L29 L91 L92 L93 L99 L101 L135 L154 L155 L156 | L99 L100 L101 L135 | L10 L11 L16 L17 A3 L21 L27 L28 L31 L32 L55 L62 L126 | L8 L29 L101 L135 L136 | A2 L25 L28 | L89 L90 L91 L92 L93 L94 L123 L155 | L8 L14 L25 L29 L96 L108 | A3 L27 L28 | L89 L90 L94 L123 L155 | L10 L31 L56 L126 L128 L129 | L8 L29 L106 L138 L139 | L10 L31 L55 L56 L58 L69 L70 L71 L116 L117 L119 L126 L128 L143 L144 L145 | L8 L29 L103 L105 L106 L113 L114 L139 L151 L152 L153 | L56 L57 L58 L128 | L106 L107 L114 L139 | L10 L31 L58 L126 L127 L128 | L8 L29 L34 L114 L139 | L50 L51 L52 L69 L70 L71 L116 L117 L118 L119 L144 | L10 L16 L27 L31 L55 L64 L83 L126 | L50 L51 L52 L118 L144 | L8 L14 L25 L29 L34 L110 | L102 L104 L112 L124 L151 | L102 L103 L104 L105 L112 L113 L124 L151 | L8 L29 L34 L37 L139 L140 | L10 L31 L86 L132 L133 | L10 L31 L78 L81 L85 L86 L88 L132 L148 L149 L150 | L10 L31 L35 L38 L132 L134 | L10 L31 L35 L88 L132 | L10 L16 L27 L31 L35 L77 | L86 L87 L88 L132 | L78 L79 L80 L81 L84 L85 L122 L149 | L79 L80 L84 L122 L149 bodies 10
extrude "Extrusion11" add sketch "Skizze2" along normal blind 0.2 from surface at 6.2 contours L11 L17 L19 L20 L21 L22 L28 L32 bodies 10
extrude "Extrusion20" add sketch "Skizze2" along normal up to surface (1.6136 mm away) from surface at 4.6864 contours L8 L14 L25 L29 L97 L98 | L8 L29 L92 L155 L156 | L8 L29 L89 L92 L123 L155 | L8 L14 L25 L29 L95 L98 | L8 L29 L89 L94 L123 L155 | L8 L14 L25 L29 L95 L96 | L8 L29 L93 L94 L123 L155 | L8 L29 L93 L154 L155 | L10 L16 L27 L31 L42 L55 L61 L62 L63 L68 L126 L142 | L8 L14 L25 L29 L108 L109 | L10 L31 L55 L63 L69 L126 L142 L144 L145 | L10 L16 L27 L31 L41 L42 L43 L44 L49 L55 L61 L63 L68 L126 L142 | L8 L14 L25 L29 L109 L111 | L8 L29 L103 L151 L152 | L10 L31 L50 L55 L63 L68 L69 L118 L126 L142 L144 | L10 L16 L27 L31 L44 L55 L61 L63 L64 L68 L126 L142 | L10 L31 L43 L49 L50 L52 L55 L63 L68 L118 L126 L142 L144 | L8 L14 L25 L29 L110 L111 | L8 L29 L102 L103 L124 L151 | L8 L29 L102 L112 L124 L151 | L10 L31 L52 L55 L63 L68 L71 L118 L126 L142 L144 | L8 L29 L112 L113 L124 L151 | L10 L31 L55 L63 L71 L126 L142 L143 L144 | L10 L16 L27 L31 L82 L83 | L8 L29 L113 L151 L153 | L10 L16 L27 L31 L76 L82 | L10 L31 L85 L148 L149 | L10 L16 L27 L31 L76 L77 | L10 L31 L79 L84 L122 L149 | L10 L31 L84 L85 L122 L149 | L10 L31 L78 L79 L122 L149 | L10 L31 L78 L149 L150 bodies 10
extrude "Extrusion21" add sketch "Skizze2" along normal blind 2.2414 from surface at 2.445 contours L8 L14 L25 L29 L95 L98 | L10 L16 L27 L31 L41 L42 L43 L44 L49 L55 L61 L63 L68 L126 L142 | L8 L14 L25 L29 L109 L111 | L10 L16 L27 L31 L76 L82 bodies 9
chamfer "Fase19" distance 2.2414 angle 45 16 edges at (31.8532, 2.445, 15.8) (29.3532, 2.445, 15.8) (13.25, 2.445, 15.8) (10.75, 2.445, 15.8) (31.8532, 2.445, -0.6) (13.25, 2.445, -0.6) (29.3532, 2.445, -0.6) (10.75, 2.445, -0.6) (29.2118, 2.445, 15.75) (31.9946, 2.445, 15.75) (10.6086, 2.445, 15.75) (13.3914, 2.445, 15.75) (31.9946, 2.445, -0.55) (29.2118, 2.445, -0.55) (10.6086, 2.445, -0.55) (13.3914, 2.445, -0.55) on bodies 9 10
extrude "Extrusion23" cut sketch "Skizze2" against normal blind 1.5414 from surface at 4.6864 contours L8 L29 L89 L92 L123 L155 | L8 L29 L89 L94 L123 L155 | L89 L90 L91 L92 L93 L94 L123 L155 | L8 L29 L93 L94 L123 L155 | L89 L90 L94 L123 L155 | L10 L31 L50 L55 L63 L68 L69 L118 L126 L142 L144 | L10 L31 L43 L49 L50 L52 L55 L63 L68 L118 L126 L142 L144 | L8 L29 L102 L103 L124 L151 | L8 L29 L102 L112 L124 L151 | L50 L51 L52 L69 L70 L71 L116 L117 L118 L119 L144 | L10 L31 L52 L55 L63 L68 L71 L118 L126 L142 L144 | L50 L51 L52 L118 L144 | L8 L29 L112 L113 L124 L151 | L102 L104 L112 L124 L151 | L102 L103 L104 L105 L112 L113 L124 L151 | L10 L31 L79 L84 L122 L149 | L10 L31 L84 L85 L122 L149 | L10 L31 L78 L79 L122 L149 | L78 L79 L80 L81 L84 L85 L122 L149 | L79 L80 L84 L122 L149 bodies 10
extrude "Extrusion22" add sketch "Skizze2" against normal blind 1.5 from surface at 4.6864 contours L8 L29 L89 L94 L123 L155 | L89 L90 L94 L123 L155 | L10 L31 L43 L49 L50 L52 L55 L63 L68 L118 L126 L142 L144 | L8 L29 L102 L112 L124 L151 | L50 L51 L52 L118 L144 | L102 L104 L112 L124 L151 | L10 L31 L79 L84 L122 L149 | L79 L80 L84 L122 L149 bodies 9
chamfer "Fase16" distance 0.5 angle 45 40 edges at (12, 4.6864, 14.7) (10.7086, 3.9157, 14.7) (13.2914, 3.9157, 14.7) (30.6032, 4.6864, 14.7) (29.3118, 3.9157, 14.7) (31.8946, 3.9157, 14.7) (10.7086, 3.9157, 0.5) (12, 4.6864, 0.5) (13.2914, 3.9157, 0.5) (29.3118, 3.9157, 0.5) (30.6032, 4.6864, 0.5) (31.8946, 3.9157, 0.5) (13.7056, 4.3725, 1.5) (10.2944, 4.3725, 1.5) (10.2944, 4.3725, 13.7) (13.7056, 4.3725, 13.7) (28.8976, 4.3725, 13.7) (32.3089, 4.3725, 13.7) (28.8976, 4.3725, 1.5) (32.3089, 4.3725, 1.5) (13.25, 3.9364, 14.8) (10.75, 3.9364, 14.8) (12, 4.6864, 14.8) (29.3532, 3.9364, 14.8) (31.8532, 3.9364, 14.8) (30.6032, 4.6864, 14.8) (29.3532, 3.9364, 0.4) (31.8532, 3.9364, 0.4) (30.6032, 4.6864, 0.4) (10.75, 3.9364, 0.4) (12, 4.6864, 0.4) (13.25, 3.9364, 0.4) (12, 3.1864, 0.4) (12, 4.6864, 0.4) (12, 4.6864, 14.8) (12, 3.1864, 14.8) (30.6032, 3.1864, 14.8) (30.6032, 4.6864, 14.8) (30.6032, 3.1864, 0.4) (30.6032, 4.6864, 0.4) on bodies 9 10
chamfer "Fase23" distance 0.5 angle 45 4 edges at (30.6032, 3.145, 14.7) (12, 3.145, 14.7) (30.6032, 3.145, 0.5) (12, 3.145, 0.5) on bodies 10
chamfer "Fase20" distance 1.0858 angle 45 4 edges at (12, 2.445, 13.7) (30.6032, 2.445, 13.7) (12, 2.445, 1.5) (30.6032, 2.445, 1.5) on bodies 10
chamfer "Fase21" distance 0.5858 angle 45 8 edges at (7.3672, 2.445, 15.0429) (16.6328, 2.445, 15.0429) (25.9704, 2.445, 15.0429) (35.2361, 2.445, 15.0429) (35.2361, 2.445, 0.1571) (25.9704, 2.445, 0.1571) (16.6328, 2.445, 0.1571) (7.3672, 2.445, 0.1571) on bodies 10
chamfer "Fase24" distance 1.05 angle 45 2 edges at (12, 6.3, 13.7) (12, 6.3, 1.5) on bodies 10
chamfer "Fase25" distance 1.55 angle 45 4 edges at (15.1692, 6.3, 14.2) (15.1692, 6.3, 1) (8.8308, 6.3, 1) (8.8308, 6.3, 14.2) on bodies 10
chamfer "Fase7" distance 1.49 distance2 2.98 1 edges at (35, 7.3, 7.6) measured on face at (35, 7.7967, 4.7) on bodies 10
chamfer "Fase22" distance 2.98 distance2 1.49 1 edges at (35.2361, 6.3, 7.6) measured on face at (20.3426, 6.3, 8.1624) on bodies 10
chamfer "Fase32" distance 2.0958 angle 30 1 edges at (-0.1, -1.41, 7.6) measured on face at (14.8, -1.41, 5.0333) on bodies 9
chamfer "Fase33" distance 2.8132 angle 30 1 edges at (-1.1, -2.41, 7.6) measured on face at (29.3667, -2.41, 4.7) on bodies 9
chamfer "Fase27" distance 0.6444 angle 45 9 edges at (3.6336, 6.3, -0.1) (21.3016, 6.3, -0.1) (21.3016, 6.3, 15.3) (3.6336, 6.3, 15.3) (-0.1, 6.3, 7.6) (23.2979, -1.41, 15.3) (23.2979, -1.41, -0.1) (0.9479, -0.805, -0.1) (0.9479, -0.805, 15.3) on bodies 9 10
chamfer "Fase28" distance 1.1 angle 45 12 edges at (0.3066, -1.5979, -1.1) (23.1566, -2.41, -1.1) (23.1566, -2.41, 16.3) (0.3066, -1.5979, 16.3) (15.4603, 7.3, 16.3) (15.4603, 7.3, -1.1) (33.5103, 8.0449, 16.3) (35, 8.7899, 16.3) (39.8, 8.79, 16.3) (33.5103, 8.0449, -1.1) (35, 8.7899, -1.1) (39.8, 8.79, -1.1) on bodies 9 10
extrude "Extrusion24" cut sketch "Skizze2" against normal blind 1.41 contours L8 L9 L10 L15 L26 L29 L30 L31 L37 L38 L134 L140 bodies 9
chamfer "Fase31" distance 0.6443 angle 45 2 edges at (35.2361, -1.41, 14.9778) (35.2361, -1.41, 0.2222) on bodies 9
extrude "Extrusion25" add sketch "Skizze2" along normal blind 0.1 from surface at 6.3 contours A5 | A6 bodies 10
equation "PCB_length = 35.6 mm"
equation "PCB_width = 15.2 mm"
equation "tolerance = 0.1 mm"
equation "d4 = PCB_length"
equation "d5 = PCB_width"
equation "USB_length = 9.5 mm"
equation "USB_width = 7.75 mm"
equation "USB_height = 4.5 mm"
equation "USB_vertical_offset = 0 mm"
equation "USB_horizontal_offset = 1.46 mm"
equation "d14 = USB_length"
equation "d15 = USB_width"
equation "PCB_thickness = 1.6 mm"
equation "ISP_length = 9 mm"
equation "ISP_width = 15.24 mm"
equation "ISP_height = 9 mm"
equation "d21 = ISP_length / 2"
equation "d22 = ISP_width"
equation "d23 = ISP_length"
equation "DIP_length = 6.7 mm"
equation "DIP_width = 9.9 mm"
equation "DIP_height = 5.7 mm"
equation "DIP_offset = 12 mm"
equation "d28 = DIP_offset"
equation "d29 = DIP_length"
equation "d30 = DIP_width"
equation "d31 = DIP_length + 2 * tolerance"
equation "d32 = DIP_width + 2 * tolerance"
equation "case_thickness = 1 mm"
equation "d34 = tolerance"
equation "d35 = tolerance"
equation "d36 = PCB_width + 2 * tolerance"
equation "d37 = PCB_length + ISP_length + tolerance"
equation "d38 = tolerance + 1 mm"
equation "d39 = tolerance + 1 mm"
equation "d40 = case_thickness"
equation "d41 = case_thickness"
equation "d42 = PCB_length + ISP_length + case_thickness + tolerance"
equation "d43 = PCB_width + 2 * case_thickness + 2 * tolerance"
equation "d44 = case_thickness + tolerance + 1 mm"
equation "d45 = case_thickness + tolerance + 1 mm"
equation "d46 = case_thickness / 2"
equation "d47 = USB_width + 2 * tolerance"
equation "d48 = case_thickness"
equation "d49 = PCB_thickness"
equation "d51 = PCB_thickness - USB_vertical_offset"
equation "d52 = USB_height"
equation "d54 = PCB_thickness"
equation "d56 = ISP_height - ISP_offset + PCB_thickness"
equation "d58 = ISP_offset - PCB_thickness"
equation "d60 = PCB_thickness"
equation "d61 = DIP_height"
equation "d63 = -ISP_offset + PCB_thickness - case_thickness - tolerance"
equation "d64 = case_thickness"
equation "d67 = total_height / 2 - case_thickness"
equation "d69 = -ISP_offset + PCB_thickness - tolerance"
equation "d71 = -PCB_thickness + USB_vertical_offset + tolerance"
equation "d73 = ISP_height - ISP_offset + PCB_thickness + tolerance"
equation "d74 = case_thickness"
equation "d76 = ISP_height - ISP_offset + PCB_thickness + tolerance"
equation "d79 = USB_height - USB_vertical_offset + PCB_thickness + tolerance"
equation "d80 = DIP_height - case_thickness - USB_height + USB_vertical_offset"
equation "d82 = PCB_length + ISP_length + case_thickness + tolerance"
equation "d83 = PCB_width + 2 * case_thickness + 2 * tolerance"
equation "d84 = PCB_width + 2 * tolerance"
equation "d85 = PCB_length + ISP_length + tolerance"
equation "ISP_offset = 2.91 mm"
equation "edge_offset = 23 mm"
equation "d105 = edge_offset"
equation "d106 = PCB_width / 2 + case_thickness + tolerance"
equation "d107 = PCB_width / 2 + case_thickness + tolerance"
equation "d108 = DIP_height + PCB_thickness - case_thickness"
equation "d109 = case_thickness"
equation "d114 = case_thickness * tan(atan(1 / chamfer_ratio) / 2)"
equation "d115 = PCB_width / 2 + case_thickness + tolerance"
equation "d116 = PCB_width / 2 + case_thickness + tolerance"
equation "d117 = DIP_height + PCB_thickness - case_thickness"
equation "d118 = ISP_height - ISP_offset - DIP_height + case_thickness + tolerance"
equation "d122 = ( ISP_height - ISP_offset - DIP_height + case_thickness + tolerance )"
equation "d126 = ( ISP_height - ISP_offset - DIP_height + case_thickness + tolerance ) * chamfer_ratio"
equation "chamfer_ratio = 2"
equation "LED_offset = 29.1 mm"
equation "LED_inner_diameter = 2.8 mm"
equation "LED_spacing = 4.2 mm"
equation "d143 = LED_offset"
equation "d144 = LED_spacing / 2"
equation "d145 = LED_spacing / 2"
equation "LED_outer_diameter = 3.2 mm"
equation "d151 = LED_outer_diameter"
equation "d152 = LED_inner_diameter"
equation "d153 = LED_inner_diameter"
equation "d154 = LED_outer_diameter"
equation "d155 = PCB_thickness"
equation "d158 = PCB_thickness + tolerance + 0.6 mm"
equation "d159 = DIP_height - tolerance - 0.6 mm"
equation "d161 = DIP_height + PCB_thickness"
equation "d162 = LED_outer_diameter / 2"
equation "d164 = LED_outer_diameter / 2"
equation "d182 = case_thickness / 2"
equation "d183 = DIP_offset + tolerance"
equation "snap_length = 2.5 mm"
equation "snap_height = 1.5 mm"
equation "snap_depth = 0.5 mm"
equation "d189 = snap_length"
equation "d190 = case_thickness"
equation "d193 = case_thickness / 2 + snap_depth / 2"
equation "d194 = case_thickness / 2 + tolerance / 2"
equation "d195 = snap_length"
equation "d196 = snap_depth"
equation "d197 = snap_length + 2 * case_thickness * ( sqrt(2) - 1 ) + 2 * tolerance * ( sqrt(2) - 1 )"
equation "d198 = case_thickness + snap_depth + tolerance"
equation "d199 = snap_length + 2 * tolerance * ( sqrt(2) )"
equation "d200 = case_thickness"
equation "d201 = tolerance / 2"
equation "d202 = snap_length + 2 * tolerance * ( sqrt(2) - 1 )"
equation "d203 = snap_depth + tolerance"
equation "d205 = PCB_width + case_thickness + 2 * tolerance"
equation "d206 = tolerance / 2"
equation "d207 = snap_depth"
equation "d208 = snap_length + 2 * tolerance * ( sqrt(2) - 1 )"
equation "d212 = total_height / 2 - ISP_offset + PCB_thickness - case_thickness - tolerance + snap_offset + snap_height + ( sqrt(2) - 1 ) * tolerance"
equation "snap_offset = 0.7 mm"
equation "d217 = snap_offset + snap_height + ( sqrt(2) - 1 ) * tolerance"
equation "d220 = -snap_height"
equation "d222 = snap_depth"
equation "d224 = case_thickness / 2 - snap_depth / 2 - tolerance / 2"
equation "d225 = 2 * ( snap_offset + snap_height + tolerance * ( 2 * sqrt(2) - 1 ) + case_thickness ) + snap_length"
equation "d226 = case_thickness + tolerance"
equation "d228 = snap_offset + snap_height + tolerance * ( sqrt(2) - 1 )"
equation "d229 = total_height / 2 - ISP_offset + PCB_thickness - case_thickness - tolerance + snap_offset + snap_height + ( sqrt(2) - 1 ) * tolerance"
equation "d230 = -snap_height - ( sqrt(2) - 1 ) * tolerance"
equation "d232 = snap_depth + case_thickness * ( 2 - sqrt(2) )"
equation "d233 = case_thickness * ( 2 - sqrt(2) )"
equation "d234 = ( ISP_height - ISP_offset - DIP_height + case_thickness + tolerance ) * chamfer_ratio"
equation "d235 = ( ISP_height - ISP_offset - DIP_height + case_thickness + tolerance )"
equation "d239 = snap_depth"
equation "d240 = case_thickness / 2 + tolerance / 2"
equation "d241 = snap_length + 2 * tolerance * ( sqrt(2) )"
equation "d242 = tolerance"
equation "d243 = PCB_width / 2 - DIP_width / 2 - tolerance - case_thickness - snap_depth"
equation "d244 = PCB_width / 2 - DIP_width / 2 - tolerance - case_thickness"
equation "d246 = chamfer_depth * ( 2 - sqrt(2) )"
equation "d247 = chamfer_depth"
equation "d250 = -ISP_offset + PCB_thickness - tolerance"
equation "d252 = chamfer_depth * ( 2 - sqrt(2) ) - 0.0001 mm"
equation "d253 = DIP_height + PCB_thickness - case_thickness"
equation "d254 = layer_height"
equation "total_height = DIP_height + ISP_offset + case_thickness + tolerance"
equation "d261 = USB_length / 2 - USB_horizontal_offset"
equation "chamfer_depth = 1.1 * case_thickness"
equation "d263 = ( ISP_offset - PCB_thickness - tolerance ) * tan(overhang_angle)"
equation "d264 = ( ISP_offset - PCB_thickness - tolerance + case_thickness * ( sqrt(2) - 1 ) ) * tan(overhang_angle)"
equation "overhang_angle = 60 deg"
equation "d266 = 90 deg - overhang_angle"
equation "d267 = 90 deg - overhang_angle"
equation "layer_height = 0.1 mm"
named bodies: "PCB", "USB plug", "DIP switches", "Bottom", "Top", "ISP header", "Green LED", "Red LED", "Optical fiber red", "Optical fiber green"
